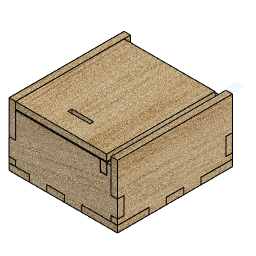
pinautomaat v6 v16 (Autodesk Fusion 360 design; units mm, degrees)
Autodesk Fusion 360 part; units mm, degrees
sketch "Sketch3" plane through (0, 0, 0) normal (0, 0, 1) x (1, 0, 0)
  line L0 (100.1763, -83.206) -> (100.1763, -67.2061)
  line L1 (100.1763, -67.2061) -> (106.1763, -67.2061)
  line L2 (106.1763, -67.2061) -> (106.1763, -51.1467)
  line L3 (106.1763, -51.1467) -> (100.1763, -51.1467)
  line L4 (100.1763, -51.1467) -> (100.1763, -35.1468)
  line L5 (100.1763, -35.1468) -> (106.1763, -35.1468)
  line L6 (106.1763, -35.1468) -> (106.1763, -6.1764)
  line L7 (106.1763, -6.1764) -> (73.2061, -6.1764)
  line L8 (73.2061, -6.1764) -> (73.2061, -12.1768)
  line L9 (73.2061, -12.1768) -> (57.2063, -12.1768)
  line L10 (57.2063, -12.1768) -> (57.2063, -6.1764)
  line L11 (57.2063, -6.1764) -> (40.8823, -6.1764)
  line L12 (40.8823, -6.1764) -> (40.8823, -12.1768)
  line L13 (40.8823, -12.1768) -> (24.8824, -12.1768)
  line L14 (24.8824, -12.1768) -> (24.8824, -6.1764)
  line L15 (24.8824, -6.1764) -> (6.1764, -6.1764)
  line L16 (6.1764, -6.1764) -> (6.1764, -35.1468)
  line L17 (6.1764, -35.1468) -> (12.1768, -35.1468)
  line L18 (12.1768, -35.1468) -> (12.1768, -51.1467)
  line L19 (12.1768, -51.1467) -> (6.1764, -51.1467)
  line L20 (6.1764, -51.1467) -> (6.1764, -67.2061)
  line L21 (6.1764, -67.2061) -> (12.1768, -67.2061)
  line L22 (12.1768, -67.2061) -> (12.1768, -83.206)
  line L23 (12.1768, -83.206) -> (6.1764, -83.206)
  line L24 (6.1764, -83.206) -> (6.1764, -112.1764)
  line L25 (6.1764, -112.1764) -> (24.8824, -112.1764)
  line L26 (24.8824, -112.1764) -> (24.8824, -106.1763)
  line L27 (24.8824, -106.1763) -> (40.8823, -106.1763)
  line L28 (40.8823, -106.1763) -> (40.8823, -112.1764)
  line L29 (40.8823, -112.1764) -> (57.2063, -112.1764)
  line L30 (57.2063, -112.1764) -> (57.2063, -106.1763)
  line L31 (57.2063, -106.1763) -> (73.2061, -106.1763)
  line L32 (73.2061, -106.1763) -> (73.2061, -112.1764)
  line L33 (73.2061, -112.1764) -> (106.1763, -112.1764)
  line L34 (106.1763, -112.1764) -> (106.1763, -83.206)
  line L35 (106.1763, -83.206) -> (100.1763, -83.206)
  line L36 (92.1757, -35.1468) -> (98.1757, -35.1468)
  line L37 (98.1757, -35.1468) -> (98.1757, -51.1467)
  line L38 (98.1757, -51.1467) -> (92.1757, -51.1467)
  line L39 (92.1757, -51.1467) -> (92.1757, -35.1468)
  line L40 (92.1757, -67.2061) -> (98.1757, -67.2061)
  line L41 (98.1757, -67.2061) -> (98.1757, -83.206)
  line L42 (98.1757, -83.206) -> (92.1757, -83.206)
  line L43 (92.1757, -83.206) -> (92.1757, -67.2061)
  line L44 (16.0401, -28.2864) -> (14.6649, -30.668)
  line L45 (14.6649, -30.668) -> (16.0401, -33.0496)
  line L46 (16.0401, -33.0496) -> (18.79, -33.0496)
  line L47 (18.79, -33.0496) -> (20.1651, -30.668)
  line L48 (20.1651, -30.668) -> (18.79, -28.2864)
  line L49 (18.79, -28.2864) -> (16.0401, -28.2864)
  line L50 (16.0401, -33.0496) -> (14.6649, -30.668)
  line L51 (14.6649, -30.668) -> (16.0401, -28.2864)
  line L52 (16.0401, -28.2864) -> (18.79, -28.2864)
  line L53 (18.79, -28.2864) -> (20.1651, -30.668)
  line L54 (20.1651, -30.668) -> (18.79, -33.0496)
  line L55 (18.79, -33.0496) -> (16.0401, -33.0496)
  line L56 (21.1313, -80.3217) -> (19.7562, -82.7033)
  line L57 (19.7562, -82.7033) -> (21.1313, -85.0848)
  line L58 (21.1313, -85.0848) -> (23.8812, -85.0848)
  line L59 (23.8812, -85.0848) -> (25.2564, -82.7033)
  line L60 (25.2564, -82.7033) -> (23.8812, -80.3217)
  line L61 (23.8812, -80.3217) -> (21.1313, -80.3217)
  line L62 (21.1313, -85.0848) -> (19.7562, -82.7033)
  line L63 (19.7562, -82.7033) -> (21.1313, -80.3217)
  line L64 (21.1313, -80.3217) -> (23.8812, -80.3217)
  line L65 (23.8812, -80.3217) -> (25.2564, -82.7033)
  line L66 (25.2564, -82.7033) -> (23.8812, -85.0848)
  line L67 (23.8812, -85.0848) -> (21.1313, -85.0848)
  line L68 (49.0007, -80.3217) -> (47.6256, -82.7033)
  line L69 (47.6256, -82.7033) -> (49.0007, -85.0848)
  line L70 (49.0007, -85.0848) -> (51.7506, -85.0848)
  line L71 (51.7506, -85.0848) -> (53.1257, -82.7033)
  line L72 (53.1257, -82.7033) -> (51.7506, -80.3217)
  line L73 (51.7506, -80.3217) -> (49.0007, -80.3217)
  line L74 (49.0007, -85.0848) -> (47.6256, -82.7033)
  line L75 (47.6256, -82.7033) -> (49.0007, -80.3217)
  line L76 (49.0007, -80.3217) -> (51.7506, -80.3217)
  line L77 (51.7506, -80.3217) -> (53.1257, -82.7033)
  line L78 (53.1257, -82.7033) -> (51.7506, -85.0848)
  line L79 (51.7506, -85.0848) -> (49.0007, -85.0848)
  line L80 (63.8385, -29.5518) -> (62.4637, -31.9334)
  line L81 (62.4637, -31.9334) -> (63.8385, -34.315)
  line L82 (63.8385, -34.315) -> (66.5884, -34.315)
  line L83 (66.5884, -34.315) -> (67.9635, -31.9334)
  line L84 (67.9635, -31.9334) -> (66.5884, -29.5518)
  line L85 (66.5884, -29.5518) -> (63.8385, -29.5518)
  line L86 (63.8385, -34.315) -> (62.4637, -31.9334)
  line L87 (62.4637, -31.9334) -> (63.8385, -29.5518)
  line L88 (63.8385, -29.5518) -> (66.5884, -29.5518)
  line L89 (66.5884, -29.5518) -> (67.9635, -31.9334)
  line L90 (67.9635, -31.9334) -> (66.5884, -34.315)
  line L91 (66.5884, -34.315) -> (63.8385, -34.315)
extrude "Extrude3" add sketch "Sketch3" along normal blind 6 makes body 1
copy_body "Body->Comp6" bodies 1 removing the originals makes body 2 in component "Component'''''"
sketch "Sketch4" plane through (0, 0, 0) normal (1, 0, 0) x (0, 1, 0)
  line L0 (248.229, -84.3405) -> (248.229, -54.3414)
  line L1 (248.229, -54.3414) -> (246.2291, -54.3414)
  line L2 (246.2291, -54.3414) -> (246.2291, -64.3416)
  line L3 (246.2291, -64.3416) -> (240.2291, -64.3416)
  line L4 (240.2291, -64.3416) -> (240.2291, -54.3414)
  line L5 (240.2291, -54.3414) -> (160.2291, -54.3414)
  line L6 (160.2291, -54.3414) -> (160.2291, -84.3405)
  line L7 (160.2291, -84.3405) -> (154.2295, -84.3405)
  line L8 (154.2295, -84.3405) -> (154.2295, -100.3407)
  line L9 (154.2295, -100.3407) -> (160.2291, -100.3407)
  line L10 (160.2291, -100.3407) -> (160.2291, -105.3409)
  line L11 (160.2291, -105.3409) -> (172.957, -105.3409)
  line L12 (172.957, -105.3409) -> (172.957, -111.341)
  line L13 (172.957, -111.341) -> (188.9561, -111.341)
  line L14 (188.9561, -111.341) -> (188.9561, -105.3409)
  line L15 (188.9561, -105.3409) -> (205.259, -105.3409)
  line L16 (205.259, -105.3409) -> (205.259, -111.341)
  line L17 (205.259, -111.341) -> (221.2578, -111.341)
  line L18 (221.2578, -111.341) -> (221.2578, -105.3409)
  line L19 (221.2578, -105.3409) -> (248.229, -105.3409)
  line L20 (248.229, -105.3409) -> (248.229, -100.341)
  line L21 (248.229, -100.341) -> (254.229, -100.341)
  line L22 (254.229, -100.341) -> (254.229, -84.3405)
  line L23 (254.229, -84.3405) -> (248.229, -84.3405)
  line L24 (248.2293, -226.2722) -> (248.2293, -221.2719)
  line L25 (248.2293, -221.2719) -> (221.2581, -221.2719)
  line L26 (221.2581, -221.2719) -> (221.2581, -215.2722)
  line L27 (221.2581, -215.2722) -> (205.2594, -215.2722)
  line L28 (205.2594, -215.2722) -> (205.2594, -221.2719)
  line L29 (205.2594, -221.2719) -> (205.0533, -221.2719)
  line L30 (205.0533, -221.2719) -> (205.0533, -235.6673)
  line L31 (205.0533, -235.6673) -> (194.1568, -235.6673)
  line L32 (194.1568, -235.6673) -> (194.1568, -221.2719)
  line L33 (194.1568, -221.2719) -> (188.9561, -221.2719)
  line L34 (188.9561, -221.2719) -> (188.9561, -215.2722)
  line L35 (188.9561, -215.2722) -> (172.957, -215.2722)
  line L36 (172.957, -215.2722) -> (172.957, -221.2719)
  line L37 (172.957, -221.2719) -> (174.8278, -221.2719)
  line L38 (174.8278, -221.2719) -> (174.8278, -235.2722)
  line L39 (174.8278, -235.2722) -> (166.1487, -235.2722)
  line L40 (166.1487, -235.2722) -> (166.1487, -221.2719)
  line L41 (166.1487, -221.2719) -> (160.2295, -221.2719)
  line L42 (160.2295, -221.2719) -> (160.2295, -226.2725)
  line L43 (160.2295, -226.2725) -> (154.2298, -226.2725)
  line L44 (154.2298, -226.2725) -> (154.2298, -242.2727)
  line L45 (154.2298, -242.2727) -> (160.2295, -242.2727)
  line L46 (160.2295, -242.2727) -> (160.2295, -272.2718)
  line L47 (160.2295, -272.2718) -> (240.2294, -272.2718)
  line L48 (240.2294, -272.2718) -> (240.2294, -262.2716)
  line L49 (240.2294, -262.2716) -> (246.2295, -262.2716)
  line L50 (246.2295, -262.2716) -> (246.2295, -272.2718)
  line L51 (246.2295, -272.2718) -> (248.2293, -272.2718)
  line L52 (248.2293, -272.2718) -> (248.2293, -242.2727)
  line L53 (248.2293, -242.2727) -> (254.2294, -242.2727)
  line L54 (254.2294, -242.2727) -> (254.2294, -226.2722)
  line L55 (254.2294, -226.2722) -> (248.2293, -226.2722)
  line L56 (287.9326, -112.3993) -> (287.9326, -118.3993)
  line L57 (287.9326, -118.3993) -> (271.9338, -118.3993)
  line L58 (271.9338, -118.3993) -> (271.9338, -112.3993)
  line L59 (271.9338, -112.3993) -> (266.9329, -112.3993)
  line L60 (266.9329, -112.3993) -> (266.9329, -141.3697)
  line L61 (266.9329, -141.3697) -> (260.8626, -141.3697)
  line L62 (260.8626, -141.3697) -> (260.8626, -157.3695)
  line L63 (260.8626, -157.3695) -> (266.9329, -157.3695)
  line L64 (266.9329, -157.3695) -> (266.9329, -173.4286)
  line L65 (266.9329, -173.4286) -> (260.8626, -173.4286)
  line L66 (260.8626, -173.4286) -> (260.8626, -189.4292)
  line L67 (260.8626, -189.4292) -> (266.9329, -189.4292)
  line L68 (266.9329, -189.4292) -> (266.9329, -218.3992)
  line L69 (266.9329, -218.3992) -> (271.9338, -218.3992)
  line L70 (271.9338, -218.3992) -> (271.9338, -212.3992)
  line L71 (271.9338, -212.3992) -> (287.9326, -212.3992)
  line L72 (287.9326, -212.3992) -> (287.9326, -218.3992)
  line L73 (287.9326, -218.3992) -> (318.9329, -218.3992)
  line L74 (318.9329, -218.3992) -> (318.9329, -112.3993)
  line L75 (318.9329, -112.3993) -> (287.9326, -112.3993)
  line L76 (149.2447, -173.429) -> (149.2447, -157.3406)
  line L77 (149.2447, -157.3406) -> (155.2444, -157.3406)
  line L78 (155.2444, -157.3406) -> (155.2444, -141.3401)
  line L79 (155.2444, -141.3401) -> (149.2447, -141.3401)
  line L80 (149.2447, -141.3401) -> (149.2447, -112.3993)
  line L81 (149.2447, -112.3993) -> (144.2438, -112.3993)
  line L82 (144.2438, -112.3993) -> (144.2438, -118.3993)
  line L83 (144.2438, -118.3993) -> (128.2446, -118.3993)
  line L84 (128.2446, -118.3993) -> (128.2446, -112.3993)
  line L85 (128.2446, -112.3993) -> (97.2444, -112.3993)
  line L86 (97.2444, -112.3993) -> (97.2444, -218.3992)
  line L87 (97.2444, -218.3992) -> (128.2446, -218.3992)
  line L88 (128.2446, -218.3992) -> (128.2446, -212.3992)
  line L89 (128.2446, -212.3992) -> (144.2438, -212.3992)
  line L90 (144.2438, -212.3992) -> (144.2438, -218.3992)
  line L91 (144.2438, -218.3992) -> (149.2447, -218.3992)
  line L92 (149.2447, -218.3992) -> (149.2447, -189.4292)
  line L93 (149.2447, -189.4292) -> (155.2448, -189.4292)
  line L94 (155.2448, -189.4292) -> (155.2448, -173.429)
  line L95 (155.2448, -173.429) -> (149.2447, -173.429)
extrude "Extrude4" add sketch "Sketch4" along normal blind 6 separate body makes body 3 at (0, 201.9057, -74.6746) makes body 4 at (0, 201.8374, -260.0703) makes body 5 at (0, 301.5996, -168.0757) makes body 6 at (0, 114.5778, -168.0758)
copy_body "Body->Comp7" bodies 3 removing the originals makes body 7 in component "Component''''''"
copy_body "Body->Comp8" bodies 6 removing the originals makes body 8 in component "Component'''''''"
copy_body "Body->Comp9" bodies 4 removing the originals makes body 9 in component "Component''''''''"
copy_body "Body->Comp10" bodies 5 removing the originals makes body 10 in component "Component'''''''''"
move_body "Move1" bodies 8 to x (-1, 0, 0) y (0, 1, 0) z (0, 0, -1) at (0, 0, -330.7985) in component "Component'''''''"
delete_face "DeleteFace1" 1 faces at (-6, 114.5778, -162.7227) on bodies 8 in component "Component'''''''"
move_body "Move2" bodies 8 to x (1, 0, 0) y (0, 0, 1) z (0, -1, 0) at (0, 31.8445, -256.6431) in component "Component'''''''"
move_body "Move1'" bodies 9 to x (1, 0, 0) y (0, 1, 0) z (0, 0, 1) at (115, 0, 0) in component "Component''''''''"
move_body "Move1''" bodies 7 to x (1, 0, 0) y (0, 1, 0) z (0, 0, 1) at (100, 0, 0) in component "Component''''''"
sketch "Sketch5" plane through (0, 0, 0) normal (0, 0, 1) x (1, 0, 0)
  line L0 (100.1759, 49.8236) -> (6.1764, 49.8236)
  line L1 (6.1764, 49.8236) -> (0.1764, 49.8236)
  line L2 (0.1764, 49.8236) -> (0.1764, 39.8234)
  line L3 (0.1764, 39.8234) -> (6.1764, 39.8234)
  line L4 (6.1764, 39.8234) -> (6.1764, 4.8237)
  line L5 (6.1764, 4.8237) -> (29.4078, 4.8237)
  line L6 (29.4078, 4.8237) -> (29.4078, -1.1763)
  line L7 (29.4078, -1.1763) -> (45.408, -1.1763)
  line L8 (45.408, -1.1763) -> (45.408, 4.8237)
  line L9 (45.408, 4.8237) -> (61.458, 4.8237)
  line L10 (61.458, 4.8237) -> (61.458, -1.1763)
  line L11 (61.458, -1.1763) -> (77.4578, -1.1763)
  line L12 (77.4578, -1.1763) -> (77.4578, 4.8237)
  line L13 (77.4578, 4.8237) -> (100.1759, 4.8237)
  line L14 (100.1759, 4.8237) -> (100.1759, 39.8234)
  line L15 (100.1759, 39.8234) -> (106.176, 39.8234)
  line L16 (106.176, 39.8234) -> (106.176, 49.8236)
  line L17 (106.176, 49.8236) -> (100.1759, 49.8236)
  line L18 (92.9983, 36.4915) -> (95.9984, 36.4915)
  line L19 (95.9984, 36.4915) -> (95.9984, 16.4915)
  line L20 (95.9984, 16.4915) -> (92.9983, 16.4915)
  line L21 (92.9983, 16.4915) -> (92.9983, 36.4915)
  line L22 (57.1294, 14.4288) -> (55.7543, 12.0472)
  line L23 (55.7543, 12.0472) -> (57.1294, 9.6656)
  line L24 (57.1294, 9.6656) -> (59.8793, 9.6656)
  line L25 (59.8793, 9.6656) -> (61.2544, 12.0472)
  line L26 (61.2544, 12.0472) -> (59.8793, 14.4288)
  line L27 (59.8793, 14.4288) -> (57.1294, 14.4288)
  line L28 (57.1294, 9.6656) -> (55.7543, 12.0472)
  line L29 (55.7543, 12.0472) -> (57.1294, 14.4284)
  line L30 (57.1294, 14.4284) -> (59.8793, 14.4284)
  line L31 (59.8793, 14.4284) -> (61.2544, 12.0472)
  line L32 (61.2544, 12.0472) -> (59.8793, 9.6656)
  line L33 (59.8793, 9.6656) -> (57.1294, 9.6656)
  line L34 (57.1294, 48.6443) -> (55.7543, 46.2627)
  line L35 (55.7543, 46.2627) -> (57.1294, 43.8811)
  line L36 (57.1294, 43.8811) -> (59.8793, 43.8811)
  line L37 (59.8793, 43.8811) -> (61.2544, 46.2627)
  line L38 (61.2544, 46.2627) -> (59.8793, 48.6443)
  line L39 (59.8793, 48.6443) -> (57.1294, 48.6443)
  line L40 (57.1294, 43.8811) -> (55.7543, 46.2627)
  line L41 (55.7543, 46.2627) -> (57.1294, 48.6443)
  line L42 (57.1294, 48.6443) -> (59.8793, 48.6443)
  line L43 (59.8793, 48.6443) -> (61.2544, 46.2627)
  line L44 (61.2544, 46.2627) -> (59.8793, 43.8811)
  line L45 (59.8793, 43.8811) -> (57.1294, 43.8811)
  line L46 (19.2941, 43.8818) -> (17.9189, 41.5002)
  line L47 (17.9189, 41.5002) -> (19.2941, 39.1186)
  line L48 (19.2941, 39.1186) -> (22.044, 39.1186)
  line L49 (22.044, 39.1186) -> (23.4191, 41.5002)
  line L50 (23.4191, 41.5002) -> (22.044, 43.8818)
  line L51 (22.044, 43.8818) -> (19.2941, 43.8818)
  line L52 (19.2941, 39.1186) -> (17.9189, 41.5002)
  line L53 (17.9189, 41.5002) -> (19.2941, 43.8818)
  line L54 (19.2941, 43.8818) -> (22.044, 43.8818)
  line L55 (22.044, 43.8818) -> (23.4191, 41.5002)
  line L56 (23.4191, 41.5002) -> (22.044, 39.1186)
  line L57 (22.044, 39.1186) -> (19.2941, 39.1186)
  line L58 (19.2941, 18.8731) -> (17.9189, 16.4911)
  line L59 (17.9189, 16.4911) -> (19.2941, 14.1095)
  line L60 (19.2941, 14.1095) -> (22.044, 14.1095)
  line L61 (22.044, 14.1095) -> (23.4191, 16.4911)
  line L62 (23.4191, 16.4911) -> (22.044, 18.8731)
  line L63 (22.044, 18.8731) -> (19.2941, 18.8731)
  line L64 (19.2941, 14.1095) -> (17.9189, 16.4911)
  line L65 (17.9189, 16.4911) -> (19.2941, 18.8727)
  line L66 (19.2941, 18.8727) -> (22.044, 18.8727)
  line L67 (22.044, 18.8727) -> (23.4191, 16.4911)
  line L68 (23.4191, 16.4911) -> (22.044, 14.1095)
  line L69 (22.044, 14.1095) -> (19.2941, 14.1095)
extrude "Extrude5" add sketch "Sketch5" along normal blind 6 separate body makes body 11
copy_body "Body->Comp11" bodies 11 removing the originals makes body 12 in component "Component''''''''''"
sketch "Sketch6" plane through (0, 0, 0) normal (1, 0, 0) x (0, 1, 0)
  line L0 (250.0215, -79.5766) -> (250.0215, -55.5775)
  line L1 (250.0215, -55.5775) -> (248.0216, -55.5775)
  line L2 (248.0216, -55.5775) -> (248.0216, -65.5777)
  line L3 (248.0216, -65.5777) -> (242.0215, -65.5777)
  line L4 (242.0215, -65.5777) -> (242.0215, -55.5775)
  line L5 (242.0215, -55.5775) -> (162.0216, -55.5775)
  line L6 (162.0216, -55.5775) -> (162.0216, -79.5769)
  line L7 (162.0216, -79.5769) -> (156.0216, -79.5769)
  line L8 (156.0216, -79.5769) -> (156.0216, -95.5768)
  line L9 (156.0216, -95.5768) -> (162.0216, -95.5768)
  line L10 (162.0216, -95.5768) -> (162.0216, -100.5774)
  line L11 (162.0216, -100.5774) -> (174.7494, -100.5774)
  line L12 (174.7494, -100.5774) -> (174.7494, -106.5771)
  line L13 (174.7494, -106.5771) -> (190.7486, -106.5771)
  line L14 (190.7486, -106.5771) -> (190.7486, -100.5774)
  line L15 (190.7486, -100.5774) -> (207.0515, -100.5774)
  line L16 (207.0515, -100.5774) -> (207.0515, -106.5771)
  line L17 (207.0515, -106.5771) -> (223.0506, -106.5771)
  line L18 (223.0506, -106.5771) -> (223.0506, -100.5774)
  line L19 (223.0506, -100.5774) -> (250.0215, -100.5774)
  line L20 (250.0215, -100.5774) -> (250.0215, -95.5771)
  line L21 (250.0215, -95.5771) -> (256.0215, -95.5771)
  line L22 (256.0215, -95.5771) -> (256.0215, -79.5766)
  line L23 (256.0215, -79.5766) -> (250.0215, -79.5766)
  line L24 (254.8623, -248.9638) -> (254.8623, -243.9636)
  line L25 (254.8623, -243.9636) -> (227.8914, -243.9636)
  line L26 (227.8914, -243.9636) -> (227.8914, -237.9635)
  line L27 (227.8914, -237.9635) -> (211.8926, -237.9635)
  line L28 (211.8926, -237.9635) -> (211.8926, -243.9636)
  line L29 (211.8926, -243.9636) -> (211.6862, -243.9636)
  line L30 (211.6862, -243.9636) -> (211.6862, -258.3586)
  line L31 (211.6862, -258.3586) -> (200.7897, -258.3586)
  line L32 (200.7897, -258.3586) -> (200.7897, -243.9636)
  line L33 (200.7897, -243.9636) -> (195.5897, -243.9636)
  line L34 (195.5897, -243.9636) -> (195.5897, -237.9635)
  line L35 (195.5897, -237.9635) -> (179.5906, -237.9635)
  line L36 (179.5906, -237.9635) -> (179.5906, -243.9636)
  line L37 (179.5906, -243.9636) -> (181.4607, -243.9636)
  line L38 (181.4607, -243.9636) -> (181.4607, -257.9635)
  line L39 (181.4607, -257.9635) -> (172.7817, -257.9635)
  line L40 (172.7817, -257.9635) -> (172.7817, -243.9636)
  line L41 (172.7817, -243.9636) -> (166.8628, -243.9636)
  line L42 (166.8628, -243.9636) -> (166.8628, -248.9642)
  line L43 (166.8628, -248.9642) -> (160.8627, -248.9642)
  line L44 (160.8627, -248.9642) -> (160.8627, -264.9637)
  line L45 (160.8627, -264.9637) -> (166.8628, -264.9637)
  line L46 (166.8628, -264.9637) -> (166.8628, -288.9631)
  line L47 (166.8628, -288.9631) -> (246.8627, -288.9631)
  line L48 (246.8627, -288.9631) -> (246.8627, -278.9633)
  line L49 (246.8627, -278.9633) -> (252.8624, -278.9633)
  line L50 (252.8624, -278.9633) -> (252.8624, -288.9631)
  line L51 (252.8624, -288.9631) -> (254.8623, -288.9631)
  line L52 (254.8623, -288.9631) -> (254.8623, -264.964)
  line L53 (254.8623, -264.964) -> (260.8626, -264.964)
  line L54 (260.8626, -264.964) -> (260.8626, -248.9638)
  line L55 (260.8626, -248.9638) -> (254.8623, -248.9638)
extrude "Extrude6" add sketch "Sketch6" along normal blind 6 separate body makes body 13 at (0, 203.6982, -73.9109) makes body 14 at (0, 208.4706, -278.7616)
copy_body "Body->Comp12" bodies 13 removing the originals makes body 15 in component "Component'''''''''''"
copy_body "Body->Comp13" bodies 14 removing the originals makes body 16 in component "Component''''''''''''"
move_body "Move1'''" bodies 15 to x (1, 0, 0) y (0, 1, 0) z (0, 0, 1) at (120, 0, 0) in component "Component'''''''''''"
move_body "Move1''''" bodies 16 to x (1, 0, 0) y (0, 1, 0) z (0, 0, 1) at (100, 0, 0) in component "Component''''''''''''"
sketch "Sketch7" plane through (0, 0, 0) normal (0, 0, 1) x (1, 0, 0)
  line L0 (0.1764, 109.8236) -> (86.176, 109.8236)
  line L1 (86.176, 109.8236) -> (86.176, 9.8241)
  line L2 (86.176, 9.8241) -> (0.1764, 9.8241)
  line L3 (0.1764, 9.8241) -> (0.1764, 109.8236)
  line L4 (33.1762, 29.7094) -> (53.1762, 29.7094)
  line L5 (53.1762, 29.7094) -> (53.1762, 26.2095)
  line L6 (53.1762, 26.2095) -> (33.1762, 26.2095)
  line L7 (33.1762, 26.2095) -> (33.1762, 29.7094)
extrude "Extrude7" add sketch "Sketch7" along normal blind 6 separate body makes body 17
copy_body "Body->Comp14" bodies 17 removing the originals makes body 18 in component "Component'''''''''''''"
move_body "Move1'''''" bodies 18 to x (1, 0, 0) y (0, 0, -1) z (0, 1, 0) at (0, 109.8236, 109.8236) in component "Component'''''''''''''"
move_body "Move2'" bodies 18 to x (1, 0, 0) y (0, 0, 1) z (0, -1, 0) at (0, 109.8236, -109.8236) in component "Component'''''''''''''"
move_body "Move3" bodies 18 to x (1, 0, 0) y (0, 1, 0) z (0, 0, 1) at (0, -2.5, 0) in component "Component'''''''''''''"
sketch "Sketch8" plane through (0, 0, 58) normal (0, 0, 1) x (-1, 0, 0)
  line L0 (-100.1763, 6.1762) -> (-100.1763, 112.1762)
  line L1 (-100.1763, 112.1762) -> (-106.1763, 112.1762)
  line L2 (-106.1763, 112.1762) -> (-106.1763, 6.1762)
  line L3 (-106.1763, 6.1762) -> (-100.1763, 6.1762)
move_body "Move4" bodies 18 to x (1, 0, 0) y (0, 0, -1) z (0, 1, 0) at (0, 107.3236, 107.3236) in component "Component'''''''''''''"
sketch "Sketch9" plane through (0, 0, 0) normal (0, 0, 1) x (1, 0, 0)
  line L0 (152.9531, -194.1754) -> (152.9531, -170.1764)
  line L1 (152.9531, -170.1764) -> (148.953, -170.1764)
  line L2 (148.953, -170.1764) -> (148.953, -180.1766)
  line L3 (148.953, -180.1766) -> (142.9533, -180.1766)
  line L4 (142.9533, -180.1766) -> (142.9533, -170.1764)
  line L5 (142.9533, -170.1764) -> (64.9536, -170.1764)
  line L6 (64.9536, -170.1764) -> (64.9536, -194.1758)
  line L7 (64.9536, -194.1758) -> (58.9536, -194.1758)
  line L8 (58.9536, -194.1758) -> (58.9536, -210.1756)
  line L9 (58.9536, -210.1756) -> (64.9536, -210.1756)
  line L10 (64.9536, -210.1756) -> (64.9536, -215.1763)
  line L11 (64.9536, -215.1763) -> (77.6815, -215.1763)
  line L12 (77.6815, -215.1763) -> (77.6815, -221.1759)
  line L13 (77.6815, -221.1759) -> (93.6806, -221.1759)
  line L14 (93.6806, -221.1759) -> (93.6806, -215.1763)
  line L15 (93.6806, -215.1763) -> (109.9835, -215.1763)
  line L16 (109.9835, -215.1763) -> (109.9835, -221.1759)
  line L17 (109.9835, -221.1759) -> (125.9823, -221.1759)
  line L18 (125.9823, -221.1759) -> (125.9823, -215.1763)
  line L19 (125.9823, -215.1763) -> (152.9531, -215.1763)
  line L20 (152.9531, -215.1763) -> (152.9531, -210.176)
  line L21 (152.9531, -210.176) -> (158.9535, -210.176)
  line L22 (158.9535, -210.176) -> (158.9535, -194.1754)
  line L23 (158.9535, -194.1754) -> (152.9531, -194.1754)
  line L24 (157.7943, -363.5627) -> (157.7943, -358.5624)
  line L25 (157.7943, -358.5624) -> (130.8234, -358.5624)
  line L26 (130.8234, -358.5624) -> (130.8234, -352.5624)
  line L27 (130.8234, -352.5624) -> (114.8243, -352.5624)
  line L28 (114.8243, -352.5624) -> (114.8243, -358.5624)
  line L29 (114.8243, -358.5624) -> (114.6179, -358.5624)
  line L30 (114.6179, -358.5624) -> (114.6179, -372.9575)
  line L31 (114.6179, -372.9575) -> (103.7217, -372.9575)
  line L32 (103.7217, -372.9575) -> (103.7217, -358.5624)
  line L33 (103.7217, -358.5624) -> (98.5214, -358.5624)
  line L34 (98.5214, -358.5624) -> (98.5214, -352.5624)
  line L35 (98.5214, -352.5624) -> (82.5223, -352.5624)
  line L36 (82.5223, -352.5624) -> (82.5223, -358.5624)
  line L37 (82.5223, -358.5624) -> (84.3927, -358.5624)
  line L38 (84.3927, -358.5624) -> (84.3927, -372.5624)
  line L39 (84.3927, -372.5624) -> (75.7137, -372.5624)
  line L40 (75.7137, -372.5624) -> (75.7137, -358.5624)
  line L41 (75.7137, -358.5624) -> (69.7944, -358.5624)
  line L42 (69.7944, -358.5624) -> (69.7944, -363.563)
  line L43 (69.7944, -363.563) -> (63.7944, -363.563)
  line L44 (63.7944, -363.563) -> (63.7944, -379.5625)
  line L45 (63.7944, -379.5625) -> (69.7944, -379.5625)
  line L46 (69.7944, -379.5625) -> (69.7944, -403.5619)
  line L47 (69.7944, -403.5619) -> (147.7941, -403.5619)
  line L48 (147.7941, -403.5619) -> (147.7941, -393.5621)
  line L49 (147.7941, -393.5621) -> (153.7941, -393.5621)
  line L50 (153.7941, -393.5621) -> (153.7941, -403.5619)
  line L51 (153.7941, -403.5619) -> (157.7943, -403.5619)
  line L52 (157.7943, -403.5619) -> (157.7943, -379.5629)
  line L53 (157.7943, -379.5629) -> (163.7947, -379.5629)
  line L54 (163.7947, -379.5629) -> (163.7947, -363.5627)
  line L55 (163.7947, -363.5627) -> (157.7943, -363.5627)
extrude "Extrude8" add sketch "Sketch9" along normal blind 6 separate body makes body 19 at (105.9635, -188.5097, 0) makes body 20 at (107.1034, -393.3605, 0)
sketch "Sketch10" plane through (0, 0, 0) normal (0, 0, 1) x (1, 0, 0)
  line L0 (100.1763, 6.794) -> (100.1763, 22.7939)
  line L1 (100.1763, 22.7939) -> (106.1763, 22.7939)
  line L2 (106.1763, 22.7939) -> (106.1763, 38.8533)
  line L3 (106.1763, 38.8533) -> (100.1763, 38.8533)
  line L4 (100.1763, 38.8533) -> (100.1763, 54.8532)
  line L5 (100.1763, 54.8532) -> (106.1763, 54.8532)
  line L6 (106.1763, 54.8532) -> (106.1763, 83.8236)
  line L7 (106.1763, 83.8236) -> (73.2061, 83.8236)
  line L8 (73.2061, 83.8236) -> (73.2061, 77.8232)
  line L9 (73.2061, 77.8232) -> (57.2063, 77.8232)
  line L10 (57.2063, 77.8232) -> (57.2063, 83.8236)
  line L11 (57.2063, 83.8236) -> (40.8823, 83.8236)
  line L12 (40.8823, 83.8236) -> (40.8823, 77.8232)
  line L13 (40.8823, 77.8232) -> (24.8824, 77.8232)
  line L14 (24.8824, 77.8232) -> (24.8824, 83.8236)
  line L15 (24.8824, 83.8236) -> (6.1764, 83.8236)
  line L16 (6.1764, 83.8236) -> (6.1764, 54.8532)
  line L17 (6.1764, 54.8532) -> (12.1768, 54.8532)
  line L18 (12.1768, 54.8532) -> (12.1768, 38.8533)
  line L19 (12.1768, 38.8533) -> (6.1764, 38.8533)
  line L20 (6.1764, 38.8533) -> (6.1764, 22.7939)
  line L21 (6.1764, 22.7939) -> (12.1768, 22.7939)
  line L22 (12.1768, 22.7939) -> (12.1768, 6.794)
  line L23 (12.1768, 6.794) -> (6.1764, 6.794)
  line L24 (6.1764, 6.794) -> (6.1764, -22.1764)
  line L25 (6.1764, -22.1764) -> (24.8824, -22.1764)
  line L26 (24.8824, -22.1764) -> (24.8824, -16.1763)
  line L27 (24.8824, -16.1763) -> (40.8823, -16.1763)
  line L28 (40.8823, -16.1763) -> (40.8823, -22.1764)
  line L29 (40.8823, -22.1764) -> (57.2063, -22.1764)
  line L30 (57.2063, -22.1764) -> (57.2063, -16.1763)
  line L31 (57.2063, -16.1763) -> (73.2061, -16.1763)
  line L32 (73.2061, -16.1763) -> (73.2061, -22.1764)
  line L33 (73.2061, -22.1764) -> (106.1763, -22.1764)
  line L34 (106.1763, -22.1764) -> (106.1763, 6.794)
  line L35 (106.1763, 6.794) -> (100.1763, 6.794)
  line L36 (90.1758, 54.8532) -> (96.1758, 54.8532)
  line L37 (96.1758, 54.8532) -> (96.1758, 38.8533)
  line L38 (96.1758, 38.8533) -> (90.1758, 38.8533)
  line L39 (90.1758, 38.8533) -> (90.1758, 54.8532)
  line L40 (90.1758, 22.7939) -> (96.1758, 22.7939)
  line L41 (96.1758, 22.7939) -> (96.1758, 6.794)
  line L42 (96.1758, 6.794) -> (90.1758, 6.794)
  line L43 (90.1758, 6.794) -> (90.1758, 22.7939)
  line L44 (16.0425, 61.7105) -> (14.6678, 59.3289)
  line L45 (14.6678, 59.3289) -> (16.0425, 56.9476)
  line L46 (16.0425, 56.9476) -> (18.7924, 56.9476)
  line L47 (18.7924, 56.9476) -> (20.1672, 59.3289)
  line L48 (20.1672, 59.3289) -> (18.7924, 61.7105)
  line L49 (18.7924, 61.7105) -> (16.0425, 61.7105)
  line L50 (16.0425, 56.9476) -> (14.6678, 59.3289)
  line L51 (14.6678, 59.3289) -> (16.0425, 61.7105)
  line L52 (16.0425, 61.7105) -> (18.7924, 61.7105)
  line L53 (18.7924, 61.7105) -> (20.1672, 59.3289)
  line L54 (20.1672, 59.3289) -> (18.7924, 56.9476)
  line L55 (18.7924, 56.9476) -> (16.0425, 56.9476)
  line L56 (21.1342, 9.6752) -> (19.7594, 7.2936)
  line L57 (19.7594, 7.2936) -> (21.1342, 4.9123)
  line L58 (21.1342, 4.9123) -> (23.8841, 4.9123)
  line L59 (23.8841, 4.9123) -> (25.2588, 7.2936)
  line L60 (25.2588, 7.2936) -> (23.8841, 9.6752)
  line L61 (23.8841, 9.6752) -> (21.1342, 9.6752)
  line L62 (21.1342, 4.9123) -> (19.7594, 7.2936)
  line L63 (19.7594, 7.2936) -> (21.1342, 9.6752)
  line L64 (21.1342, 9.6752) -> (23.8841, 9.6752)
  line L65 (23.8841, 9.6752) -> (25.2588, 7.2936)
  line L66 (25.2588, 7.2936) -> (23.8841, 4.9123)
  line L67 (23.8841, 4.9123) -> (21.1342, 4.9123)
  line L68 (49.0035, 9.6752) -> (47.6288, 7.2936)
  line L69 (47.6288, 7.2936) -> (49.0035, 4.9123)
  line L70 (49.0035, 4.9123) -> (51.7534, 4.9123)
  line L71 (51.7534, 4.9123) -> (53.1282, 7.2936)
  line L72 (53.1282, 7.2936) -> (51.7534, 9.6752)
  line L73 (51.7534, 9.6752) -> (49.0035, 9.6752)
  line L74 (49.0035, 4.9123) -> (47.6288, 7.2936)
  line L75 (47.6288, 7.2936) -> (49.0035, 9.6752)
  line L76 (49.0035, 9.6752) -> (51.7534, 9.6752)
  line L77 (51.7534, 9.6752) -> (53.1282, 7.2936)
  line L78 (53.1282, 7.2936) -> (51.7534, 4.9123)
  line L79 (51.7534, 4.9123) -> (49.0035, 4.9123)
  line L80 (63.8413, 60.4451) -> (62.4666, 58.0635)
  line L81 (62.4666, 58.0635) -> (63.8413, 55.6822)
  line L82 (63.8413, 55.6822) -> (66.5912, 55.6822)
  line L83 (66.5912, 55.6822) -> (67.966, 58.0635)
  line L84 (67.966, 58.0635) -> (66.5912, 60.4451)
  line L85 (66.5912, 60.4451) -> (63.8413, 60.4451)
  line L86 (63.8413, 55.6822) -> (62.4666, 58.0635)
  line L87 (62.4666, 58.0635) -> (63.8413, 60.4451)
  line L88 (63.8413, 60.4451) -> (66.5912, 60.4451)
  line L89 (66.5912, 60.4451) -> (67.966, 58.0635)
  line L90 (67.966, 58.0635) -> (66.5912, 55.6822)
  line L91 (66.5912, 55.6822) -> (63.8413, 55.6822)
extrude "Extrude9" add sketch "Sketch10" along normal blind 6 separate body makes body 21
copy_body "Body->Comp15" bodies 21 removing the originals makes body 22 in component "Component''''''''''''''"
copy_body "Body->Comp16" bodies 19 removing the originals makes body 23 in component "Component'''''''''''''''"
copy_body "Body->Comp17" bodies 20 removing the originals makes body 24 in component "Component''''''''''''''''"
sketch "Sketch11" plane through (0, 0, 0) normal (0, 0, 1) x (1, 0, 0)
  line L0 (0.1764, 109.8236) -> (84.1761, 109.8236)
  line L1 (84.1761, 109.8236) -> (84.1761, 9.8241)
  line L2 (84.1761, 9.8241) -> (0.1764, 9.8241)
  line L3 (0.1764, 9.8241) -> (0.1764, 109.8236)
  line L4 (32.1761, 29.7094) -> (52.1761, 29.7094)
  line L5 (52.1761, 29.7094) -> (52.1761, 26.2095)
  line L6 (52.1761, 26.2095) -> (32.1761, 26.2095)
  line L7 (32.1761, 26.2095) -> (32.1761, 29.7094)
extrude "Extrude10" add sketch "Sketch11" along normal blind 6 separate body makes body 25
copy_body "Body->Comp18" bodies 25 removing the originals makes body 26 in component "Component'''''''''''''''''"
sketch "Sketch1" plane through (0, 0, 0) normal (0, 0, 1) x (1, 0, 0)
  line L0 (100.1763, -83.206) -> (100.1763, -67.2061)
  line L1 (100.1763, -67.2061) -> (106.1763, -67.2061)
  line L2 (106.1763, -67.2061) -> (106.1763, -51.1467)
  line L3 (106.1763, -51.1467) -> (100.1763, -51.1467)
  line L4 (100.1763, -51.1467) -> (100.1763, -35.1468)
  line L5 (100.1763, -35.1468) -> (106.1763, -35.1468)
  line L6 (106.1763, -35.1468) -> (106.1763, -6.1764)
  line L7 (106.1763, -6.1764) -> (73.2061, -6.1764)
  line L8 (73.2061, -6.1764) -> (73.2061, -12.1768)
  line L9 (73.2061, -12.1768) -> (57.2063, -12.1768)
  line L10 (57.2063, -12.1768) -> (57.2063, -6.1764)
  line L11 (57.2063, -6.1764) -> (40.8823, -6.1764)
  line L12 (40.8823, -6.1764) -> (40.8823, -12.1768)
  line L13 (40.8823, -12.1768) -> (24.8824, -12.1768)
  line L14 (24.8824, -12.1768) -> (24.8824, -6.1764)
  line L15 (24.8824, -6.1764) -> (6.1764, -6.1764)
  line L16 (6.1764, -6.1764) -> (6.1764, -35.1468)
  line L17 (6.1764, -35.1468) -> (12.1768, -35.1468)
  line L18 (12.1768, -35.1468) -> (12.1768, -51.1467)
  line L19 (12.1768, -51.1467) -> (6.1764, -51.1467)
  line L20 (6.1764, -51.1467) -> (6.1764, -67.2061)
  line L21 (6.1764, -67.2061) -> (12.1768, -67.2061)
  line L22 (12.1768, -67.2061) -> (12.1768, -83.206)
  line L23 (12.1768, -83.206) -> (6.1764, -83.206)
  line L24 (6.1764, -83.206) -> (6.1764, -112.1764)
  line L25 (6.1764, -112.1764) -> (24.8824, -112.1764)
  line L26 (24.8824, -112.1764) -> (24.8824, -106.1763)
  line L27 (24.8824, -106.1763) -> (40.8823, -106.1763)
  line L28 (40.8823, -106.1763) -> (40.8823, -112.1764)
  line L29 (40.8823, -112.1764) -> (57.2063, -112.1764)
  line L30 (57.2063, -112.1764) -> (57.2063, -106.1763)
  line L31 (57.2063, -106.1763) -> (73.2061, -106.1763)
  line L32 (73.2061, -106.1763) -> (73.2061, -112.1764)
  line L33 (73.2061, -112.1764) -> (106.1763, -112.1764)
  line L34 (106.1763, -112.1764) -> (106.1763, -83.206)
  line L35 (106.1763, -83.206) -> (100.1763, -83.206)
  line L36 (92.1757, -35.1468) -> (98.1757, -35.1468)
  line L37 (98.1757, -35.1468) -> (98.1757, -51.1467)
  line L38 (98.1757, -51.1467) -> (92.1757, -51.1467)
  line L39 (92.1757, -51.1467) -> (92.1757, -35.1468)
  line L40 (92.1757, -67.2061) -> (98.1757, -67.2061)
  line L41 (98.1757, -67.2061) -> (98.1757, -83.206)
  line L42 (98.1757, -83.206) -> (92.1757, -83.206)
  line L43 (92.1757, -83.206) -> (92.1757, -67.2061)
  line L44 (16.0401, -28.2864) -> (14.6649, -30.668)
  line L45 (14.6649, -30.668) -> (16.0401, -33.0496)
  line L46 (16.0401, -33.0496) -> (18.79, -33.0496)
  line L47 (18.79, -33.0496) -> (20.1651, -30.668)
  line L48 (20.1651, -30.668) -> (18.79, -28.2864)
  line L49 (18.79, -28.2864) -> (16.0401, -28.2864)
  line L50 (16.0401, -33.0496) -> (14.6649, -30.668)
  line L51 (14.6649, -30.668) -> (16.0401, -28.2864)
  line L52 (16.0401, -28.2864) -> (18.79, -28.2864)
  line L53 (18.79, -28.2864) -> (20.1651, -30.668)
  line L54 (20.1651, -30.668) -> (18.79, -33.0496)
  line L55 (18.79, -33.0496) -> (16.0401, -33.0496)
  line L56 (21.1313, -80.3217) -> (19.7562, -82.7033)
  line L57 (19.7562, -82.7033) -> (21.1313, -85.0848)
  line L58 (21.1313, -85.0848) -> (23.8812, -85.0848)
  line L59 (23.8812, -85.0848) -> (25.2564, -82.7033)
  line L60 (25.2564, -82.7033) -> (23.8812, -80.3217)
  line L61 (23.8812, -80.3217) -> (21.1313, -80.3217)
  line L62 (21.1313, -85.0848) -> (19.7562, -82.7033)
  line L63 (19.7562, -82.7033) -> (21.1313, -80.3217)
  line L64 (21.1313, -80.3217) -> (23.8812, -80.3217)
  line L65 (23.8812, -80.3217) -> (25.2564, -82.7033)
  line L66 (25.2564, -82.7033) -> (23.8812, -85.0848)
  line L67 (23.8812, -85.0848) -> (21.1313, -85.0848)
  line L68 (49.0007, -80.3217) -> (47.6256, -82.7033)
  line L69 (47.6256, -82.7033) -> (49.0007, -85.0848)
  line L70 (49.0007, -85.0848) -> (51.7506, -85.0848)
  line L71 (51.7506, -85.0848) -> (53.1257, -82.7033)
  line L72 (53.1257, -82.7033) -> (51.7506, -80.3217)
  line L73 (51.7506, -80.3217) -> (49.0007, -80.3217)
  line L74 (49.0007, -85.0848) -> (47.6256, -82.7033)
  line L75 (47.6256, -82.7033) -> (49.0007, -80.3217)
  line L76 (49.0007, -80.3217) -> (51.7506, -80.3217)
  line L77 (51.7506, -80.3217) -> (53.1257, -82.7033)
  line L78 (53.1257, -82.7033) -> (51.7506, -85.0848)
  line L79 (51.7506, -85.0848) -> (49.0007, -85.0848)
  line L80 (63.8385, -29.5518) -> (62.4637, -31.9334)
  line L81 (62.4637, -31.9334) -> (63.8385, -34.315)
  line L82 (63.8385, -34.315) -> (66.5884, -34.315)
  line L83 (66.5884, -34.315) -> (67.9635, -31.9334)
  line L84 (67.9635, -31.9334) -> (66.5884, -29.5518)
  line L85 (66.5884, -29.5518) -> (63.8385, -29.5518)
  line L86 (63.8385, -34.315) -> (62.4637, -31.9334)
  line L87 (62.4637, -31.9334) -> (63.8385, -29.5518)
  line L88 (63.8385, -29.5518) -> (66.5884, -29.5518)
  line L89 (66.5884, -29.5518) -> (67.9635, -31.9334)
  line L90 (67.9635, -31.9334) -> (66.5884, -34.315)
  line L91 (66.5884, -34.315) -> (63.8385, -34.315)
sketch "Sketch2" plane through (0, 0, 0) normal (0, 1, 0) x (1, 0, 0)
  line L0 (279.8184, -111.341) -> (279.8184, -117.341)
  line L1 (279.8184, -117.341) -> (263.8196, -117.341)
  line L2 (263.8196, -117.341) -> (263.8196, -111.341)
  line L3 (263.8196, -111.341) -> (258.819, -111.341)
  line L4 (258.819, -111.341) -> (258.819, -139.7233)
  line L5 (258.819, -139.7233) -> (252.819, -139.7233)
  line L6 (252.819, -139.7233) -> (252.819, -155.7231)
  line L7 (252.819, -155.7231) -> (258.819, -155.7231)
  line L8 (258.819, -155.7231) -> (258.819, -171.7822)
  line L9 (258.819, -171.7822) -> (252.819, -171.7822)
  line L10 (252.819, -171.7822) -> (252.819, -187.7828)
  line L11 (252.819, -187.7828) -> (258.819, -187.7828)
  line L12 (258.819, -187.7828) -> (258.819, -217.3409)
  line L13 (258.819, -217.3409) -> (263.8196, -217.3409)
  line L14 (263.8196, -217.3409) -> (263.8196, -211.3409)
  line L15 (263.8196, -211.3409) -> (279.8184, -211.3409)
  line L16 (279.8184, -211.3409) -> (279.8184, -217.3409)
  line L17 (279.8184, -217.3409) -> (310.819, -217.3409)
  line L18 (310.819, -217.3409) -> (310.819, -111.341)
  line L19 (310.819, -111.341) -> (279.8184, -111.341)
  line L20 (156.9885, -155.6572) -> (156.9885, -139.6573)
  line L21 (156.9885, -139.6573) -> (150.9885, -139.6573)
  line L22 (150.9885, -139.6573) -> (150.9885, -111.341)
  line L23 (150.9885, -111.341) -> (145.9886, -111.341)
  line L24 (145.9886, -111.341) -> (145.9886, -117.341)
  line L25 (145.9886, -117.341) -> (129.9895, -117.341)
  line L26 (129.9895, -117.341) -> (129.9895, -111.341)
  line L27 (129.9895, -111.341) -> (98.9888, -111.341)
  line L28 (98.9888, -111.341) -> (98.9888, -217.3409)
  line L29 (98.9888, -217.3409) -> (129.9895, -217.3409)
  line L30 (129.9895, -217.3409) -> (129.9895, -211.3409)
  line L31 (129.9895, -211.3409) -> (145.9886, -211.3409)
  line L32 (145.9886, -211.3409) -> (145.9886, -217.3409)
  line L33 (145.9886, -217.3409) -> (150.9885, -217.3409)
  line L34 (150.9885, -217.3409) -> (150.9885, -187.7828)
  line L35 (150.9885, -187.7828) -> (156.9885, -187.7828)
  line L36 (156.9885, -187.7828) -> (156.9885, -171.7822)
  line L37 (156.9885, -171.7822) -> (150.9885, -171.7822)
  line L38 (150.9885, -171.7822) -> (150.9885, -155.6572)
  line L39 (150.9885, -155.6572) -> (156.9885, -155.6572)
  line L40 (248.229, -84.3405) -> (248.229, -54.3414)
  line L41 (248.229, -54.3414) -> (246.2291, -54.3414)
  line L42 (246.2291, -54.3414) -> (246.2291, -64.3416)
  line L43 (246.2291, -64.3416) -> (240.2291, -64.3416)
  line L44 (240.2291, -64.3416) -> (240.2291, -54.3414)
  line L45 (240.2291, -54.3414) -> (160.2291, -54.3414)
  line L46 (160.2291, -54.3414) -> (160.2291, -84.3405)
  line L47 (160.2291, -84.3405) -> (154.2295, -84.3405)
  line L48 (154.2295, -84.3405) -> (154.2295, -100.3407)
  line L49 (154.2295, -100.3407) -> (160.2291, -100.3407)
  line L50 (160.2291, -100.3407) -> (160.2291, -105.3409)
  line L51 (160.2291, -105.3409) -> (172.957, -105.3409)
  line L52 (172.957, -105.3409) -> (172.957, -111.341)
  line L53 (172.957, -111.341) -> (188.9561, -111.341)
  line L54 (188.9561, -111.341) -> (188.9561, -105.3409)
  line L55 (188.9561, -105.3409) -> (205.259, -105.3409)
  line L56 (205.259, -105.3409) -> (205.259, -111.341)
  line L57 (205.259, -111.341) -> (221.2578, -111.341)
  line L58 (221.2578, -111.341) -> (221.2578, -105.3409)
  line L59 (221.2578, -105.3409) -> (248.229, -105.3409)
  line L60 (248.229, -105.3409) -> (248.229, -100.341)
  line L61 (248.229, -100.341) -> (254.229, -100.341)
  line L62 (254.229, -100.341) -> (254.229, -84.3405)
  line L63 (254.229, -84.3405) -> (248.229, -84.3405)
  line L64 (248.2293, -226.2722) -> (248.2293, -221.2719)
  line L65 (248.2293, -221.2719) -> (221.2581, -221.2719)
  line L66 (221.2581, -221.2719) -> (221.2581, -215.2722)
  line L67 (221.2581, -215.2722) -> (205.2594, -215.2722)
  line L68 (205.2594, -215.2722) -> (205.2594, -221.2719)
  line L69 (205.2594, -221.2719) -> (205.0533, -221.2719)
  line L70 (205.0533, -221.2719) -> (205.0533, -235.6673)
  line L71 (205.0533, -235.6673) -> (194.1568, -235.6673)
  line L72 (194.1568, -235.6673) -> (194.1568, -221.2719)
  line L73 (194.1568, -221.2719) -> (188.9561, -221.2719)
  line L74 (188.9561, -221.2719) -> (188.9561, -215.2722)
  line L75 (188.9561, -215.2722) -> (172.957, -215.2722)
  line L76 (172.957, -215.2722) -> (172.957, -221.2719)
  line L77 (172.957, -221.2719) -> (174.8278, -221.2719)
  line L78 (174.8278, -221.2719) -> (174.8278, -235.2722)
  line L79 (174.8278, -235.2722) -> (166.1487, -235.2722)
  line L80 (166.1487, -235.2722) -> (166.1487, -221.2719)
  line L81 (166.1487, -221.2719) -> (160.2295, -221.2719)
  line L82 (160.2295, -221.2719) -> (160.2295, -226.2725)
  line L83 (160.2295, -226.2725) -> (154.2298, -226.2725)
  line L84 (154.2298, -226.2725) -> (154.2298, -242.2727)
  line L85 (154.2298, -242.2727) -> (160.2295, -242.2727)
  line L86 (160.2295, -242.2727) -> (160.2295, -272.2718)
  line L87 (160.2295, -272.2718) -> (240.2294, -272.2718)
  line L88 (240.2294, -272.2718) -> (240.2294, -262.2716)
  line L89 (240.2294, -262.2716) -> (246.2295, -262.2716)
  line L90 (246.2295, -262.2716) -> (246.2295, -272.2718)
  line L91 (246.2295, -272.2718) -> (248.2293, -272.2718)
  line L92 (248.2293, -272.2718) -> (248.2293, -242.2727)
  line L93 (248.2293, -242.2727) -> (254.2294, -242.2727)
  line L94 (254.2294, -242.2727) -> (254.2294, -226.2722)
  line L95 (254.2294, -226.2722) -> (248.2293, -226.2722)
extrude "Extrude1" [suppressed]
extrude "Extrude2" [suppressed]
copy_body "Body->Comp1" [suppressed] in component "Component"
copy_body "Body->Comp2" [suppressed] in component "Component'"
copy_body "Body->Comp3" [suppressed] in component "Component''"
copy_body "Body->Comp4" [suppressed] in component "Component'''"
copy_body "Body->Comp5" [suppressed] in component "Component''''"
component "Component'''''" placed x (1, 0, 0) y (0, 1, 0) z (0, 0, 1) at (3.2598, -13.3515, 2.3918)
component "Component''''''" placed x (0, -1, 0) y (1, 0, 0) z (0, 0, 1) at (-144.8035, -19.5279, 113.7328)
component "Component'''''''" placed x (1, 0, 0) y (0, -1, 0) z (0, 0, -1) at (15.4362, 124.7303, -99.0065)
component "Component''''''''" placed x (0, 1, 0) y (1, 0, 0) z (0, 0, -1) at (-144.8144, -140.5283, -212.8804)
component "Component'''''''''" placed x (1, 0, 0) y (0, 0, 1) z (0, -1, 0) at (103.4361, -237.9269, -258.541)
component "Component''''''''''" placed x (0, -1, 0) y (0, 0, 1) z (-1, 0, 0) at (99.4356, -19.0994, 3.4979)
component "Component'''''''''''" placed x (0, -1, 0) y (1, 0, 0) z (0, 0, 1) at (-146.6069, 0.4722, 108.9689)
component "Component''''''''''''" placed x (0, 1, 0) y (1, 0, 0) z (0, 0, -1) at (-151.4265, -125.5135, -235.5716)
component "Component'''''''''''''" placed x (1, 0, 0) y (0, 1, 0) z (0, 0, 1) at (15.2598, -129.337, 54.3922)
component "Component''''''''''''''" placed x (1, 0, 0) y (0, 1, 0) z (0, 0, 1) at (3.2598, -103.3513, 2.3216)
component "Component'''''''''''''''" placed x (1, 0, 0) y (0, 0, 1) z (0, -1, 0) at (-49.5389, -119.5276, 223.4975)
component "Component''''''''''''''''" placed x (1, 0, 0) y (0, 0, -1) z (0, 1, 0) at (-54.3797, -25.5281, -350.2408)
component "Component'''''''''''''''''" placed x (1, 0, 0) y (0, 1, 0) z (0, 0, 1) at (15.2384, -135.3517, 54.3211)
